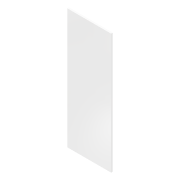
# Autodesk Inventor part: 00_Sample_Doubleslit
Saved by Autodesk Inventor 2022 (Build 260153000, 153)
## iProperties
Created: 2022-10-12
Part Number: 00_Sample_Doubleslit
Material: Generisch
Document SubType Name: Modeling
Designer: UC2
Density: 1 g/cm^3
Appearance: Polycarbonat - klar
Author: UC2
Autodesk Inventor part; units mm, degrees
ref_plane "YZ Plane" through (0, 0, 0) normal (1, 0, 0) x (0, 1, 0)
ref_plane "XZ Plane" through (0, 0, 0) normal (0, 1, 0) x (-1, 0, 0)
ref_plane "XY Plane" through (0, 0, 0) normal (0, 0, 1) x (1, 0, 0)
sketch "Skizze1" plane through (0, 0, 0) normal (0, 0, 1) x (1, 0, 0)
  line L0 (13.5, -37) -> (-13.5, -37)
  line L1 (-13.5, -37) -> (-13.5, 37)
  line L2 (-13.5, 37) -> (13.5, 37)
  line L3 (13.5, 37) -> (13.5, -37)
  line L4 (13.5, -37) -> (-13.5, 37) construction
  line L5 (-13.5, -37) -> (13.5, 37) construction
  point P0 (0, 0)
  dimension "d0" = 27
  dimension "d1" = 74
  constraints: 12 end point, 2 midpoint, 2 parallel, 1 horizontal, 1 perpendicular
  measures "d0" distance of L1.end L2.end
  measures "d1" distance of L0.end L1.end
extrude "Extrusion1" add sketch "Skizze1" along normal blind 1
